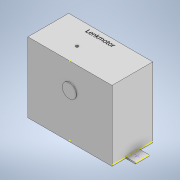
# Autodesk Inventor part: Lenkmotor1
Saved by Autodesk Inventor 2021 (Build 250183000, 183)
## iProperties
Created: 2021-01-26
Part Number: Lenkmotor1
Material: Gold
Document SubType Name: Modeling
Designer: LETPJG
Density: 19.3 g/cm^3
Appearance: Vorgabe
Author: LETPJG
Autodesk Inventor part; units mm, degrees
ref_plane "YZ Plane" through (0, 0, 0) normal (1, 0, 0) x (0, 1, 0)
ref_plane "XZ Plane" through (0, 0, 0) normal (0, 1, 0) x (-1, 0, 0)
ref_plane "XY Plane" through (0, 0, 0) normal (0, 0, 1) x (1, 0, 0)
sketch "Skizze1" plane through (0, 0, 0) normal (0, 0, 1) x (1, 0, 0)
  line L0 (30, -25) -> (-30, -25)
  line L1 (-30, -25) -> (-30, 25)
  line L2 (-30, 25) -> (30, 25)
  line L3 (30, 25) -> (30, -25)
  point P0 (0, 0)
  point P1 (-30, 0)
  point P2 (0, 25)
  dimension "d0" = 50
  dimension "d1" = 60
  constraints: 8 end point, 2 midpoint, 2 parallel, 1 horizontal, 1 horizontal alignment, 1 perpendicular, 1 vertical alignment
  measures "d0" distance of L2.end L0.start
  measures "d1" distance of L0.start L0.end
extrude "Extrusion1" add sketch "Skizze1" against normal blind 29.1
sketch "Skizze2" plane through (0, 0, 0) normal (0, 0, 1) x (1, 0, 0)
  line L0 (-30, -25) -> (30, -25) projected
  circle A0 centre (0, 6.981) radius 5
  point P0 (0, 0)
  dimension "d4" = 31.981
  dimension "d5" = 10
  constraints: 1 centre point, 1 coincident
  measures "d4" distance from line of L0 point (0, 6.981)
  measures "d5" diameter of A0
sketch "Skizze3" plane through (-30, 25, 0) normal (0, 1, 0) x (1, 0, 0)
  circle A0 centre (23.3356, 11.6912) radius 1
  point P0 (30, 0)
  dimension "d6" = 2
  constraints: 1 centre point
  measures "d6" diameter of A0
extrude "Extrusion2" cut sketch "Skizze3" against normal blind 10
sketch "Skizze4" plane through (30, -25, 0) normal (1, 0, 0) x (0, 0, -1)
  line L0 (0, 0) -> (0, 50) projected
  line L1 (0, 0) -> (29.1, 0) projected
  line L2 (29.1, 0) -> (19.4, 0)
  line L3 (9.7, 0) -> (19.4, 0)
  line L4 (19.4, 0) -> (19.4, 1)
  line L5 (19.4, 1) -> (9.7, 1)
  line L6 (9.7, 1) -> (9.7, 0)
  point P0 (0, 25)
  constraints: 10 end point, 2 parallel, 2 point on line, 1 horizontal, 1 perpendicular
extrude "Extrusion3" add sketch "Skizze4" along normal blind 7
mirror "Spiegeln1" about plane through (0, 0, 0) normal (1, 0, 0) of "Extrusion3"
sketch "Skizze5" plane through (30, -24, -9.7) normal (0, 1, 0) x (1, 0, 0)
  line L0 (7, 0) -> (7, 9.7) projected
  line L1 (0, -9.7) -> (0, 19.4) projected
  line L2 (0, -9.7) -> (0, 0) projected
  line L3 (-60, 9.7) -> (-60, 0) projected
  line L4 (-60, 9.7) -> (-67, 9.7) projected
  line L5 (-67, 9.7) -> (-67, 0) projected
  point P0 (-30, -9.7)
  point P1 (3.5, 4.7412)
  point P2 (-63.5, 4.85)
sketch "Skizze6" plane through (-30, 25, 0) normal (0, 1, 0) x (1, 0, 0)
  line L0 (17.0015, 26.6738) -> (64.1972, 26.6738) construction
  line L1 (64.1972, 26.6738) -> (64.1972, 22.3208) construction
  line L2 (64.1972, 22.3208) -> (17.0015, 22.3208) construction
  line L3 (17.0015, 22.3208) -> (17.0015, 26.6738) construction
  point P0 (30, 0)
  constraints: 2 other
extrude "Extrusion4" add sketch "Skizze2" along normal blind 0.5
